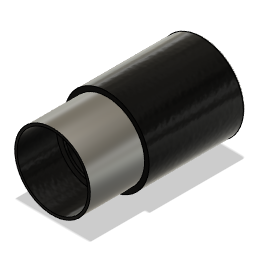
Eyepiece v2 (Autodesk Fusion 360 design; units mm, degrees)
part number: Eyepiece
Autodesk Fusion 360 part; units mm, degrees
sketch "Sketch1" plane through (0, 0, 0) normal (1, 0, 0) x (0, 0, -1)
  line L0 (0, 12.45) -> (0, 14.875)
  line L1 (0, 14.875) -> (-16.51, 14.875)
  line L2 (-16.51, 14.875) -> (-16.51, 15.875)
  line L3 (-16.51, 15.875) -> (6.35, 15.875)
  line L4 (6.35, 15.875) -> (6.35, 17.78)
  line L5 (6.35, 17.78) -> (46.99, 17.78)
  line L6 (46.99, 17.78) -> (46.99, 12.5)
  line L7 (46.99, 12.5) -> (44.99, 12.5)
  line L8 (44.99, 12.5) -> (44.99, 0)
  line L9 (44.99, 0) -> (6.35, 0)
  line L10 (6.35, 0) -> (6.35, 14.875)
  line L11 (6.35, 14.875) -> (1, 14.875)
  line L12 (1, 14.875) -> (1, 12.45)
  line L13 (1, 12.45) -> (0, 12.45)
  dimension "d532" = 15.875
  dimension "d533" = 1
  dimension "d534" = 12.45
  dimension "d535" = 14.875
  dimension "d536" = 5.35
  dimension "d537" = 16.51
  dimension "d538" = 17.78
  dimension "d539" = 40.64
  dimension "d540" = 12.5
  dimension "d541" = 2
  dimension "d545" = 0
  dimension "d546" = 0
  dimension "d547" = 0
  dimension "d548" = 0
  constraint perpendicular L1 L2
  constraint perpendicular L2 L3
  constraint perpendicular L3 L4
  constraint perpendicular L4 L5
  constraint perpendicular L5 L6
  constraint perpendicular L6 L7
  constraint perpendicular L7 L8
  constraint perpendicular L9 L10
  constraint perpendicular L11 L12
  constraint horizontal L13
  constraint collinear L1 L11
  constraint horizontal L9
  constraint coincident origin L9
  constraint collinear L4 L10
  constraint coincident origin L0
  constraint vertical L0
  measures "d532" distance of origin L3
  measures "d533" distance of L0.start L12.end
  measures "d534" distance of origin L13
  measures "d535" distance of L9.end L10.end
  measures "d536" distance of L10.end L11.end
  measures "d537" distance of L0.end L1.end
  measures "d538" distance of L5 L9
  measures "d539" distance of L4.end L5.end
  measures "d540" distance of L7.end L8.end
  measures "d541" distance of L6.end L7.end
revolve "Revolve1" add sketch "Sketch1" angle 360 about axis through (0, 0, 1.75) along (0, 0, 1)
fillet "Fillet1" radius 1 2 edges at (-16.5768, 6.4295, -46.99) (-11.6541, 4.5202, -46.99)
equation "d532 = 1.25 in / 2"
